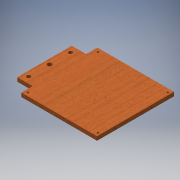
# Autodesk Inventor part: Byggeplade Holder
Saved by Autodesk Inventor 2016 (Build 200138000, 138)
## iProperties
Created: 2015-05-11
Part Number: Byggeplade Holder
Material: Wood (Cherry)
Document SubType Name: Modeling
Designer: Mathias Lyngklip Kjeldgaard
Density: 0.63 g/cm^3
Appearance: Cherry - Natural Low Gloss
Mass: 515.19 g
Surface Area: 1512.55 cm^2
Volume: 817.761 cm^3
Author: Mathias Lyngklip Kjeldgaard
Title: Byggeplade Holder
Revision Number: 1
Autodesk Inventor part; units mm, degrees
ref_plane "YZ Plane" through (0, 0, 0) normal (1, 0, 0) x (0, 1, 0)
ref_plane "XZ Plane" through (0, 0, 0) normal (0, 1, 0) x (-1, 0, 0)
ref_plane "XY Plane" through (0, 0, 0) normal (0, 0, 1) x (1, 0, 0)
sketch "Sketch1" plane through (0, 0, 0) normal (0, 0, 1) x (1, 0, 0)
  line L0 (-173, 120) -> (173, 120)
  line L1 (173, 120) -> (173, -120)
  line L2 (173, -120) -> (-173, -120)
  line L3 (-173, -120) -> (-173, 120)
  point P0 (0, 0)
  dimension "d0" = 173
  dimension "d1" = 240
  dimension "d2" = 346
  dimension "d3" = 120
  constraints: 8 end point, 2 parallel, 1 horizontal, 1 perpendicular
  measures "d0" distance from line of L1 point (0, 0)
  measures "d1" distance of L0.end L1.end
  measures "d2" distance of L1.end L2.end
  measures "d3" distance from line of point (0, 0) L2
extrude "Plade tykkelse" add sketch "Sketch1" along normal blind 12
sketch "Sketch2" plane through (0, 0, 12) normal (0, 0, 1) x (1, 0, 0)
  line L0 (5, 88) -> (-145, 88) projected
  line L1 (5, 88) -> (5, 100) projected
  line L2 (-145, 100) -> (5, 100) projected
  line L3 (-145, 88) -> (-145, 100) projected
  line L4 (5, -100) -> (-145, -100) projected
  line L5 (5, -100) -> (5, -88) projected
  line L6 (-145, -88) -> (5, -88) projected
  line L7 (-145, -100) -> (-145, -88) projected
  circle A0 centre (-115, 109) radius 3
  circle A1 centre (103, 109) radius 3
  circle A2 centre (-115, -109) radius 3
  circle A3 centre (103, -109) radius 3
  circle A4 centre (-157, 65) radius 6
  circle A5 centre (-157, 0) radius 7
  circle A6 centre (-157, -65) radius 6
  point P0 (0, 0)
  dimension "d22" = 6
  dimension "d23" = 6
  dimension "d24" = 6
  dimension "d25" = 6
  dimension "d26" = 218
  dimension "d27" = 218
  dimension "d28" = 218
  dimension "d29" = 218
  dimension "d36" = 12
  dimension "d37" = 14
  dimension "d38" = 12
  dimension "d39" = 130
  dimension "d40" = 65
  dimension "d41" = 157
  dimension "d42" = 157
  dimension "d43" = 157
  dimension "d44" = 0
  dimension "d45" = 109
  dimension "d46" = 109
  dimension "d64" = 115
  dimension "d65" = 115
  constraints: 7 centre point
  measures "d22" diameter of A0
  measures "d23" diameter of A1
  measures "d24" diameter of A3
  measures "d25" diameter of A2
  measures "d26" distance of A1.centre A0.centre
  measures "d27" distance of A2.centre A0.centre
  measures "d28" distance of A1.centre A3.centre
  measures "d29" distance of A3.centre A2.centre
  measures "d36" diameter of A4
  measures "d37" diameter of A5
  measures "d38" diameter of A6
  measures "d39" distance of A6.centre A4.centre
  measures "d40" vertical distance of point (0, 0) A6.centre
  measures "d41" horizontal distance of point (0, 0) A6.centre
  measures "d42" horizontal distance of point (0, 0) A4.centre
  measures "d43" distance of point (0, 0) A5.centre
  measures "d44" vertical distance of point (0, 0) A5.centre
  measures "d45" vertical distance of point (0, 0) A3.centre
  measures "d46" vertical distance of point (0, 0) A2.centre
  measures "d64" horizontal distance of point (0, 0) A2.centre
  measures "d65" horizontal distance of point (0, 0) A0.centre
extrude "Monteringshuller & -udskæringer" cut sketch "Sketch2" against normal blind 14 contours A0 | A1 | A2 | A3 | A4 | A5 | A6
sketch "Sketch3" plane through (0, 0, 12) normal (0, 0, 1) x (1, 0, 0)
  circle A0 centre (103, -109) radius 3 projected
  line L0 (-173, -120) -> (173, -120) projected
  line L1 (173, -120) -> (173, 120) projected
  line L2 (173, 120) -> (111, 120)
  line L3 (111, 120) -> (111, -120)
  line L4 (111, -120) -> (173, -120)
  line L5 (173, -120) -> (173, 120)
  point P0 (0, 0)
  dimension "d47" = 8
  constraints: 8 end point, 2 parallel, 1 horizontal, 1 perpendicular, 1 point on line
  measures "d47" distance from line of L3 A0.centre
extrude "Sidste længde tilpasning" cut sketch "Sketch3" against normal blind 16 contours L3 L2 L1 L0
sketch "Sketch5" plane through (0, 0, 12) normal (0, 0, 1) x (1, 0, 0)
  line L0 (111, 120) -> (-173, 120) construction
  line L1 (-173, 120) -> (-173, -120) construction
  line L2 (-173, -120) -> (111, -120) construction
  circle A0 centre (-157, 0) radius 7 construction
  circle A1 centre (-157, 65) radius 6 construction
  circle A2 centre (-115, -109) radius 3 construction
  circle A3 centre (-115, 109) radius 3 construction
  circle A4 centre (103, 109) radius 3 construction
  circle A5 centre (103, -109) radius 3 construction
  circle A6 centre (-157, -65) radius 6 construction
  line L3 (-173, -120) -> (-173, 120) projected
  line L4 (-173, -120) -> (-125, -120)
  line L5 (-125, -120) -> (-125, -85)
  line L6 (-125, -85) -> (-173, -85)
  line L7 (-173, -85) -> (-173, -120)
  line L8 (-173, 120) -> (-128, 120)
  line L9 (-128, 120) -> (-128, 85)
  line L10 (-128, 85) -> (-173, 85)
  line L11 (-173, 85) -> (-173, 120)
  line L12 (111, -120) -> (111, 120) projected
  point P0 (0, 0)
  dimension "d58" = 48
  dimension "d59" = 35
  dimension "d60" = 45
  dimension "d61" = 35
  constraints: 16 end point, 4 parallel, 2 horizontal, 2 perpendicular
  measures "d58" distance of L6.end L5.end
  measures "d59" distance of L5.end L4.end
  measures "d60" distance of L9.end L10.end
  measures "d61" distance of L8.end L9.end
extrude "CutOff" cut sketch "Sketch5" against normal up to surface (12 mm away)
equation "\"d0\" = 0.5 * d2"
equation "\"d3\" = 0.5 * d1"
equation "\"d23\" = d22"
equation "\"d24\" = d22"
equation "\"d25\" = d22"
equation "\"d26\" = d29"
equation "\"d27\" = d28"
equation "\"d40\" = 0.5 * d39"
equation "\"d42\" = d41"
equation "\"d43\" = d41"
equation "\"d45\" = 0.5 * d28"
equation "\"d46\" = 0.5 * d27"
equation "\"d65\" = d64"
body "Solid1"
